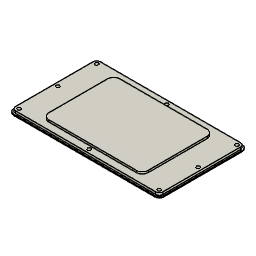
Display Mount PRO - Blank (Autodesk Fusion 360 design; units mm, degrees)
Autodesk Fusion 360 part; units mm, degrees
note: some values were not read from the file. Set by a fixed rule: which sketch regions a step uses.
sketch "Sketch1" plane through (0, 0, 0) normal (0, 0, 1) x (1, 0, 0)
  circle A0 centre (-93.5, 51.75) radius 2.3
  circle A1 centre (93.5, 51.75) radius 2.3
  circle A2 centre (-93.5, -51.75) radius 2.3
  circle A3 centre (93.5, -51.75) radius 2.3
  line L0 (-93.5, 51.75) -> (93.5, 51.75) construction
  line L1 (93.5, 51.75) -> (93.5, -51.75) construction
  line L2 (93.5, -51.75) -> (-93.5, -51.75) construction
  line L3 (-93.5, -51.75) -> (-93.5, 51.75) construction
  circle A4 centre (-93.5, 0) radius 2.3
  circle A5 centre (0, 51.75) radius 2.3
  circle A6 centre (93.5, 0) radius 2.3
  circle A7 centre (0, -51.75) radius 2.3
  line L4 (0, 87.0412) -> (0, 82.962)
  line L5 (0, 82.962) -> (0, -82.962) construction
  line L6 (-123.3001, 0) -> (123.3001, 0) construction
  circle A8 centre (93.5, -51.75) radius 4.9
  circle A9 centre (-93.5, -51.75) radius 4.9
  circle A10 centre (-93.5, 51.75) radius 4.9
  circle A11 centre (93.5, 51.75) radius 4.9
  line L7 (-93.4999, 56.65) -> (93.5, 56.65)
  line L8 (98.4, 51.75) -> (98.4, -51.75)
  line L9 (-93.5, -56.65) -> (-65.5347, -56.65)
  line L10 (-65.5347, -56.65) -> (93.5, -56.65)
  line L11 (-98.4, 51.75) -> (-98.4, -51.75)
  point P0 (0, 51.75)
  point P1 (93.5, 0)
  point P2 (0, -51.75)
  point P3 (-93.5, 0)
  dimension "d23" = 4.6
  dimension "d24" = 4.6
  dimension "d25" = 4.6
  dimension "d26" = 4.6
  dimension "d92" = 4.6
  dimension "d93" = 4.6
  dimension "d94" = 4.6
  dimension "d95" = 4.6
  dimension "d178" = 187
  dimension "d179" = 103.5
  dimension "d180" = 9.8
  dimension "d181" = 9.8
  dimension "d182" = 9.8
  dimension "d183" = 9.8
  constraint coincident A0.centre L0.start
  constraint coincident A3.centre L1.end
  constraint coincident A2.centre L2.end
  constraint midpoint L0 P0
  constraint midpoint L1 P1
  constraint midpoint L2 P2
  constraint midpoint L3 P3
  constraint coincident P3 A4.centre
  constraint coincident P0 A5.centre
  constraint coincident P1 A6.centre
  constraint coincident P2 A7.centre
  constraint midpoint origin L6
  constraint midpoint origin L5
  constraint symmetric A0.centre A1.centre L5
  constraint vertical A0.centre P3
  constraint symmetric A0.centre A2.centre L6
  constraint coincident P1 L6
  constraint parallel L0 L2
  constraint parallel L1 L3
  constraint coincident P0 L5
  constraint concentric A3 A8
  constraint concentric A2 A9
  constraint concentric A0 A10
  constraint concentric A1 A11
  constraint coincident A10 L7.start
  constraint coincident A11 L7.end
  constraint parallel L0 L7
  constraint tangent A11 L7
  constraint coincident A11 L8.start
  constraint coincident A8 L8.end
  constraint vertical L8
  constraint tangent A8 L8
  constraint coincident A9 L9.start
  constraint tangent A9 L9
  constraint perpendicular L5 L9
  constraint coincident A8 L10.end
  constraint tangent A8 L10
  constraint perpendicular L5 L10
  constraint coincident A10 L11.start
  constraint coincident A9 L11.end
  constraint tangent A9 L11
  constraint tangent A10 L11
  measures "d23" diameter of A0
  measures "d24" diameter of A1
  measures "d25" diameter of A2
  measures "d26" diameter of A3
  measures "d92" diameter of A4
  measures "d93" diameter of A7
  measures "d94" diameter of A6
  measures "d95" diameter of A5
  measures "d178" distance of A0.centre A1.centre
  measures "d179" distance of A0.centre A2.centre
  measures "d180" diameter of A8
  measures "d181" diameter of A9
  measures "d182" diameter of A10
  measures "d183" diameter of A11
extrude "Extrude1" add sketch "Sketch1" along normal blind 3
sketch "Sketch6" plane through (0, 0, 3) normal (0, 0, 1) x (-1, 0, 0)
  circle A0 centre (-93.5, 51.75) radius 2.3
  circle A1 centre (-93.5, -51.75) radius 2.3
  circle A2 centre (93.5, -51.75) radius 2.3
  circle A3 centre (93.5, 51.75) radius 2.3
  line L0 (0, -100) -> (0, 100) construction
  line L1 (148.8555, 0) -> (144.6445, 0)
  line L2 (144.6445, 0) -> (-144.6445, 0) construction
  line L3 (66.4, -47.3125) -> (-66.4, -47.3125)
  line L4 (-66.4, -47.3125) -> (-66.4, 47.3125)
  line L5 (-66.4, 47.3125) -> (66.4, 47.3125)
  line L6 (66.4, 47.3125) -> (66.4, -47.3125)
  circle A4 centre (0, 51.75) radius 2.3
  circle A5 centre (93.5, 0) radius 2.3
  circle A6 centre (0, -51.75) radius 2.3
  circle A7 centre (-93.5, 0) radius 2.3
  arc A8 (-93.5, 56.65) -> (-98.4, 51.75) centre (-93.5, 51.75) ccw
  arc A9 (-98.4, -51.75) -> (-93.5, -56.65) centre (-93.5, -51.75) ccw
  arc A10 (93.4999, -56.65) -> (98.4, -51.75) centre (93.5, -51.75) ccw
  arc A11 (98.4, 51.75) -> (93.5, 56.65) centre (93.5, 51.75) ccw
  line L7 (-93.5, -56.65) -> (93.4999, -56.65)
  line L8 (98.4, -51.75) -> (98.4, 51.75)
  line L9 (93.5, 56.65) -> (-93.5, 56.65)
  line L10 (-98.4, 51.75) -> (-98.4, -51.75)
  constraint vertical L0
  constraint horizontal L1
  constraint midpoint origin L2
  constraint midpoint origin L0
  constraint horizontal L3
  constraint vertical L4
  constraint horizontal L5
  constraint vertical L6
  constraint symmetric L0 L4 L6
  constraint symmetric L2 L3 L5
extrude "Extrude7" add sketch "Sketch6" along normal blind 2.6 contours L3 L4 L5 L6
fillet "Fillet2" radius 8 4 edges at (-66.4, -47.3125, 4.3) (66.4, -47.3125, 4.3) (66.4, 47.3125, 4.3) (-66.4, 47.3125, 4.3)
sketch "Sketch7" plane through (0, 0, 5.6) normal (0, 0, 1) x (-1, 0, 0)
  arc A0 (58.4, -47.3125) -> (66.4, -39.3125) centre (58.4, -39.3125) ccw
  line L0 (66.4, -39.3125) -> (66.4, 39.3125)
  arc A1 (66.4, 39.3125) -> (58.4, 47.3125) centre (58.4, 39.3125) ccw
  line L1 (58.4, 47.3125) -> (-58.4, 47.3125)
  arc A2 (-58.4, 47.3125) -> (-66.4, 39.3125) centre (-58.4, 39.3125) ccw
  line L2 (-66.4, 39.3125) -> (-66.4, -39.3125)
  arc A3 (-66.4, -39.3125) -> (-58.4, -47.3125) centre (-58.4, -39.3125) ccw
  line L3 (-58.4, -47.3125) -> (58.4, -47.3125)
  line L4 (0, -73.9327) -> (0, 73.9327) construction
  line L5 (109.5416, 0) -> (107.2442, 0)
  line L6 (107.2442, 0) -> (-107.2442, 0) construction
  line L7 (39.5, -33.25) -> (-41.5, -33.25)
  line L8 (-41.5, -33.25) -> (-41.5, 18.25)
  line L9 (-41.5, 18.25) -> (39.5, 18.25)
  line L10 (39.5, 18.25) -> (39.5, -33.25)
  line L11 (39.5, 35.05) -> (-41.5, 35.05) construction
  line L12 (46.5, -44.5) -> (-46.5, -44.5) construction
  line L13 (-46.5, -44.5) -> (-46.5, 44.5) construction
  line L14 (-46.5, 44.5) -> (46.5, 44.5) construction
  line L15 (46.5, 44.5) -> (46.5, -44.5) construction
  line L16 (39, 18.25) -> (39, 33.25) construction
  circle A4 centre (44, -39.5) radius 2.5 construction
  circle A5 centre (-44, -39.5) radius 2.5 construction
  circle A6 centre (44, -39.5) radius 1.4
  circle A7 centre (-44, -39.5) radius 1.4
  circle A8 centre (-44, -39.5) radius 3.5
  circle A9 centre (44, -39.5) radius 3.5
  line L17 (47.5, -47.3125) -> (-47.5, -47.3125)
  line L18 (-47.5, -47.3125) -> (-47.5, 47.3125)
  line L19 (-47.5, 47.3125) -> (47.5, 47.3125)
  line L20 (47.5, 47.3125) -> (47.5, -47.3125)
  line L21 (39, 27.05) -> (23, 27.05)
  line L22 (23, 27.05) -> (23, 43.05)
  line L23 (23, 43.05) -> (39, 43.05)
  line L24 (39, 43.05) -> (39, 27.05)
  line L25 (31, 27.05) -> (31, 43.05) construction
  line L26 (39, 35.05) -> (23, 35.05) construction
  line L27 (-41.5, -33.25) -> (-46, -33.25)
  line L28 (-46, -33.25) -> (-46, 14.25)
  line L29 (-46, 14.25) -> (-41.5, 14.25)
  line L30 (-41.5, 14.25) -> (-41.5, -33.25)
  line L31 (47.5, 45.5) -> (-47.5, 45.5)
  line L32 (47.5, -45.5) -> (-47.5, -45.5)
  circle A10 centre (44, 25.5) radius 2.5
  circle A11 centre (44, 25.5) radius 1.4
  circle A12 centre (-44, 25.5) radius 2.5
  circle A13 centre (-44, 25.5) radius 1.4
  circle A14 centre (44, 25.5) radius 3.5
  line L33 (47.5, 17.0503) -> (41.5251, 23.0251)
  line L34 (47.5, 33.9497) -> (41.5251, 27.9749)
  circle A15 centre (-44, 25.5) radius 3.5
  line L35 (-41.5251, 23.0251) -> (-47.5, 17.0503)
  line L36 (-41.5251, 27.9749) -> (-47.5, 33.9497)
  circle A16 centre (31, 35.05) radius 5
  line L37 (40.5, -45.5) -> (40.5, -39.5)
  line L38 (44, -36) -> (47.5, -36)
  line L39 (-44, -36) -> (-47.5, -36)
  line L40 (-40.5, -39.5) -> (-40.5, -45.5)
  line L41 (44, -39.5) -> (-44, -39.5) construction
  circle A17 centre (-1, 35.05) radius 3
  point P0 (31, 35.05)
  point P1 (-1, 35.05)
  dimension "d96" = 16.8
  dimension "d98" = 46.5
  dimension "d99" = 44.5
  dimension "d100" = 11.25
  dimension "d101" = 26.25
  dimension "d103" = 5
  dimension "d104" = 5
  dimension "d107" = 2.8
  dimension "d108" = 2.8
  dimension "d113" = 7
  dimension "d114" = 7
  dimension "d116" = 7
  dimension "d118" = 5
  dimension "d121" = 16
  dimension "d123" = 16
  dimension "d124" = 4.5
  dimension "d134" = 1
  dimension "d135" = 1
  dimension "d136" = 5
  dimension "d137" = 2.8
  dimension "d138" = 5
  dimension "d139" = 2.8
  dimension "d140" = 65
  dimension "d141" = 7
  dimension "d142" = 45
  dimension "d143" = 45
  dimension "d147" = 4
  dimension "d148" = 7
  dimension "d149" = 45
  dimension "d150" = 45
  dimension "d151" = 1
  dimension "d152" = 10
  dimension "d166" = 3.5
  dimension "d167" = 3.5
  dimension "d169" = 5
  dimension "d170" = 69
  dimension "d177" = 8.5
  dimension "d11" = 32
  dimension "d12" = 6
  constraint perpendicular L1 L4
  constraint perpendicular L0 L5
  constraint perpendicular L2 L6
  constraint midpoint origin L6
  constraint midpoint origin L4
  constraint horizontal L7
  constraint vertical L8
  constraint horizontal L9
  constraint vertical L10
  constraint perpendicular L8 L11
  constraint vertical L8.end L11.end
  constraint vertical L9.end L11.start
  constraint horizontal L12
  constraint vertical L13
  constraint horizontal L14
  constraint vertical L15
  constraint symmetric L6 L12 L14
  constraint coincident L9 L16.start
  constraint perpendicular L9 L16
  constraint horizontal A4.centre A5.centre
  constraint tangent L15 A4
  constraint concentric A4 A6
  constraint concentric A5 A7
  constraint concentric A5 A8
  constraint concentric A4 A9
  constraint horizontal L17
  constraint vertical L18
  constraint horizontal L19
  constraint vertical L20
  constraint coincident L1 L18.end
  constraint coincident L3 L17.start
  constraint tangent A8 L18
  constraint tangent A9 L20
  constraint horizontal L21
  constraint vertical L22
  constraint horizontal L23
  constraint vertical L24
  constraint midpoint L21 L25.start
  constraint midpoint L23 L25.end
  constraint midpoint L24 L26.start
  constraint midpoint L22 L26.end
  constraint coincident L25 P0
  constraint coincident L26 P0
  constraint coincident L11 P0
  constraint collinear L16 L24
  constraint horizontal L27
  constraint vertical L28
  constraint vertical L30
  constraint coincident L20 L31.start
  constraint coincident L18 L31.end
  constraint perpendicular L18 L31
  constraint coincident L20 L32.start
  constraint coincident L18 L32.end
  constraint perpendicular L18 L32
  constraint concentric A10 A11
  constraint tangent L15 A10
  constraint concentric A12 A13
  constraint tangent L13 A12
  constraint horizontal A10.centre A12.centre
  constraint concentric A11 A14
  constraint coincident L20 L33.start
  constraint coincident A14 L33.end
  constraint tangent A14 L33
  constraint coincident L20 L34.start
  constraint coincident A14 L34.end
  constraint tangent A14 L34
  constraint perpendicular L29 L30
  constraint concentric A13 A15
  constraint coincident L18 L35.end
  constraint coincident A15 L36.start
  constraint coincident L18 L36.end
  constraint tangent A15 L35
  constraint tangent A15 L36
  constraint coincident A15 L35.start
  constraint coincident P0 A16.centre
  constraint coincident A9 L37.end
  constraint tangent A9 L37
  constraint perpendicular L12 L37
  constraint coincident A9 L38.start
  constraint tangent A9 L38
  constraint perpendicular L15 L38
  constraint coincident A8 L39.start
  constraint tangent A8 L39
  constraint perpendicular L13 L39
  constraint coincident A8 L40.start
  constraint tangent A8 L40
  constraint perpendicular L12 L40
  constraint coincident L20 L38.end
  constraint coincident L32 L37.start
  constraint coincident L18 L39.end
  constraint coincident L32 L40.end
  constraint coincident A4.centre A6.centre
  constraint coincident A5.centre A7.centre
  constraint coincident L11 P1
  constraint coincident P1 A17.centre
  measures "d96" distance of L9 L11
  measures "d98" distance of L4 L13.end
  measures "d99" distance of L6 L13.end
  measures "d100" distance of L7 L12
  measures "d101" distance of L9 L14
  measures "d103" diameter of A4
  measures "d104" diameter of A5
  measures "d107" diameter of A6
  measures "d108" diameter of A7
  measures "d113" diameter of A8
  measures "d114" diameter of A9
  measures "d116" distance of L10 L15
  measures "d118" distance of L8 L13
  measures "d121" distance of L22.end L23.end
  measures "d123" distance of L21 L23
  measures "d124" distance of L8 L28
  measures "d134" distance of L14 L31
  measures "d135" distance of L12 L32
  measures "d136" diameter of A10
  measures "d137" diameter of A11
  measures "d138" diameter of A12
  measures "d139" diameter of A13
  measures "d140" distance of A4.centre A10.centre
  measures "d141" diameter of A14
  measures "d142" angle of L20 L33
  measures "d143" angle of L20 L34
  measures "d147" distance of L8.end L29.end
  measures "d148" diameter of A15
  measures "d149" angle of L18 L35
  measures "d150" angle of L18 L36
  measures "d151" distance of L13 L18
  measures "d152" diameter of A16
  measures "d166" distance of A5.centre L18
  measures "d167" distance of A4.centre L20
  measures "d169" distance of L12 L41
  measures "d177" distance of L10 P0
  measures "d11" distance of P0 P1
  measures "d12" diameter of A17
sketch "Sketch8" plane through (0, 0, 0) normal (0, 0, -1) x (1, 0, 0)
  circle A0 centre (93.5, 51.75) radius 2.3
  circle A1 centre (0, 51.75) radius 2.3
  circle A2 centre (-93.5, 0) radius 2.3
  circle A3 centre (-93.5, 51.75) radius 2.3
  circle A4 centre (93.5, -51.75) radius 2.3
  circle A5 centre (0, -51.75) radius 2.3
  circle A6 centre (-93.5, -51.75) radius 2.3
  circle A7 centre (93.5, 0) radius 2.3
  line L0 (93.5, 58.65) -> (-93.5, 58.65)
  line L1 (-100.4, 51.75) -> (-100.4, -51.75)
  line L2 (-93.5, -58.65) -> (93.5, -58.65)
  line L3 (100.4, -51.75) -> (100.4, 51.75)
  arc A8 (98.4, 51.75) -> (93.5, 56.65) centre (93.5, 51.75) ccw
  arc A9 (-93.5, 56.65) -> (-98.4, 51.75) centre (-93.5, 51.75) ccw
  arc A10 (-98.4, -51.75) -> (-93.4999, -56.65) centre (-93.5, -51.75) ccw
  arc A11 (93.5, -56.65) -> (98.4, -51.75) centre (93.5, -51.75) ccw
  line L4 (98.4, -51.75) -> (98.4, 51.75)
  line L5 (93.5, 56.65) -> (-93.5, 56.65)
  line L6 (-98.4, 51.75) -> (-98.4, -51.75)
  line L7 (-93.4999, -56.65) -> (93.5, -56.65)
  circle A12 centre (93.5, 51.75) radius 6.9
  circle A13 centre (-93.5, 51.75) radius 6.9
  circle A14 centre (-93.5, -51.75) radius 6.9
  circle A15 centre (93.5, -51.75) radius 6.9
  dimension "d184" = 2
  dimension "d185" = 2
  dimension "d186" = 2
  dimension "d187" = 2
  constraint concentric A0 A12
  constraint tangent L3 A12
  constraint tangent L0 A13
  constraint tangent L1 A13
  constraint coincident A3.centre A9.centre
  constraint tangent L1 A14
  constraint tangent L2 A14
  constraint coincident A6.centre A10.centre
  constraint tangent L2 A15
  constraint tangent L3 A15
  constraint coincident A4.centre A11.centre
  constraint coincident L0.end A13
  constraint coincident L0.start A12
  constraint coincident L2.end A15
  constraint coincident L2.start A14
  constraint coincident L1.start A13
  constraint coincident L1.end A14
  constraint coincident L3.start A15
  constraint coincident L3.end A12
  measures "d184" distance of L1 L6
  measures "d185" distance of L0 L5
  measures "d186" distance of L3 L4
  measures "d187" distance of L2 L7
extrude "Extrude15" add sketch "Sketch8" along normal blind 2.4
fillet "Fillet5" radius 1 8 edges at (100.4, 0, -2.4) (98.379, -56.629, -2.4) (0, -58.65, -2.4) (-98.379, -56.629, -2.4) (-100.4, 0, -2.4) (-98.379, 56.629, -2.4) (0, 58.65, -2.4) (98.379, 56.629, -2.4)
equation "d24 = d23"
equation "d25 = d23"
equation "d26 = d23"
equation "d92 = d23"
equation "d93 = d23"
equation "d94 = d23"
equation "d95 = d23"
equation "d98 = ( 93 / 2 ) * 1 mm"
equation "d99 = ( 89 / 2 ) * 1 mm"
equation "d108 = d107"
equation "d113 = d111"
equation "d114 = d111"
equation "d121 = d123"
equation "d137 = d107"
equation "d139 = d107"
equation "d180 = d181"
equation "d182 = d181"
equation "d183 = d181"
equation "d111 = 7 mm"
